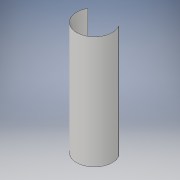
# Autodesk Inventor part: DPLX_P015_Foil_Wrap_SG
Saved by Autodesk Inventor 2018 (Build 220112000, 112)
## iProperties
Created: 2018-06-12
Part Number: DPLX_P015_Foil_Wrap_SG
Material: Generic
Document SubType Name: Modeling
Designer: DPLXuser
Density: 1 g/cm^3
Appearance: Default
Author: DPLXuser
Autodesk Inventor part; units mm, degrees
ref_plane "YZ Plane" through (0, 0, 0) normal (1, 0, 0) x (0, 1, 0)
ref_plane "XZ Plane" through (0, 0, 0) normal (0, 1, 0) x (-1, 0, 0)
ref_plane "XY Plane" through (0, 0, 0) normal (0, 0, 1) x (1, 0, 0)
sketch "Sketch1" plane through (0, 0, 0) normal (0, 1, 0) x (-1, 0, 0)
  circle A0 centre (0, 0) radius 12
  circle A1 centre (0, 0) radius 12.008
  dimension "d0" = 24
  dimension "d1" = 24.016
  constraints: 2 centre point, 2 coincident
  measures "d0" diameter of A0
  measures "d1" diameter of A1
extrude "Extrusion1" add sketch "Sketch1" along normal blind 76.2 contours A0 | A1
shell "Shell1" thickness 0.016 removed faces 2 at (3.8864, 76.2, 0.9579) at (3.8864, 0, 0.9579)
sketch "Sketch2" plane through (0, 0, 0) normal (0, 1, 0) x (-1, 0, 0)
  line L0 (0, 0) -> (10.414, 0)
  line L1 (10.414, 0) -> (10.414, -23.8671)
  line L2 (10.414, -23.8671) -> (-10.414, -23.8671)
  line L3 (-10.414, -23.8671) -> (-10.414, 0)
  line L4 (-10.414, 0) -> (0, 0)
  dimension "d5" = 10.414
  dimension "d6" = 20.828
  constraints: 10 end point, 3 perpendicular, 1 collinear, 1 horizontal, 1 point on line
  measures "d5" distance of L0.start L0.end
  measures "d6" distance of L1.end L2.end
extrude "Extrusion2" cut sketch "Sketch2" along normal blind 76.2
body "Solid1"
